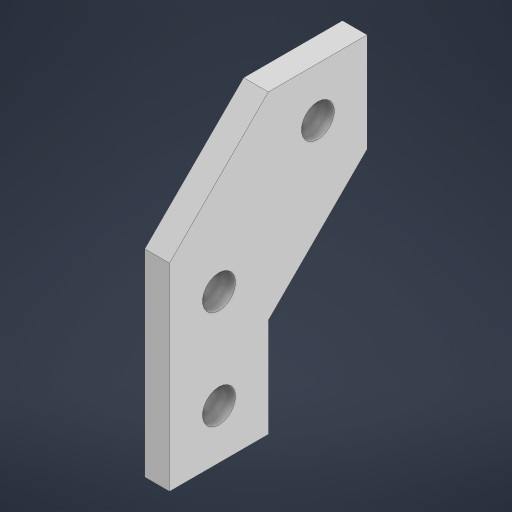
# Autodesk Inventor part: sled mounts
Saved by Autodesk Inventor 2024 (Build 280153000, 153)
## iProperties
Created: 2024-03-28
Part Number: sled mounts
Material: Generic
Document SubType Name: Modeling
Designer: Andrew
Density: 1 g/cm^3
Appearance: Default
Author: Andrew
Autodesk Inventor part; units mm, degrees
ref_plane "YZ Plane" through (0, 0, 0) normal (1, 0, 0) x (0, 1, 0)
ref_plane "XZ Plane" through (0, 0, 0) normal (0, 1, 0) x (-1, 0, 0)
ref_plane "XY Plane" through (0, 0, 0) normal (0, 0, 1) x (1, 0, 0)
sketch "Sketch1" plane through (0, 0, 0) normal (1, 0, 0) x (0, 1, 0)
  line L0 (0, 0) -> (12.7, 0)
  circle A0 centre (12.7, 0) radius 2.1209
  circle A1 centre (0, 0) radius 2.1209
  line L1 (12.7, 0) -> (12.7, 6.35)
  line L2 (12.7, 6.35) -> (19.05, 6.35)
  line L3 (19.05, 6.35) -> (-6.35, 6.35)
  line L4 (-6.35, 6.35) -> (-6.35, -6.35)
  line L5 (-6.35, -6.35) -> (19.05, -6.35)
  line L6 (19.05, -6.35) -> (19.05, 6.35)
  line L7 (19.05, -6.35) -> (19.05, -19.05)
  line L8 (19.05, -19.05) -> (31.75, -19.05)
  line L9 (31.75, -19.05) -> (31.75, -6.35)
  line L10 (31.75, -6.35) -> (19.05, 6.35)
  line L11 (19.05, -19.05) -> (6.35, -6.35)
  line L12 (19.05, -12.7) -> (25.4, -12.7)
  circle A2 centre (25.4, -12.7) radius 2.1082
  dimension "d0" = 12.7
  dimension "d1" = 4.2418
  dimension "d2" = 4.2418
  dimension "d3" = 6.35
  dimension "d4" = 6.35
  dimension "d5" = 25.4
  dimension "d6" = 12.7
  dimension "d7" = 12.7
  dimension "d8" = 4.2164
  constraints: 26 end point, 3 centre point, 3 coincident, 3 horizontal, 3 perpendicular, 2 midpoint, 2 parallel, 2 vertical
  measures "d0" distance of L0.start L0.end
  measures "d1" diameter of A0
  measures "d2" diameter of A1
  measures "d3" distance of L1.start L1.end
  measures "d4" distance of L1.end L2.end
  measures "d5" distance of L5.end L4.end
  measures "d6" distance of L5.end L7.end
  measures "d7" distance of L7.end L8.end
  measures "d8" diameter of A2
extrude "Extrusion1" add sketch "Sketch1" along normal blind 3.175
body "Solid1"
